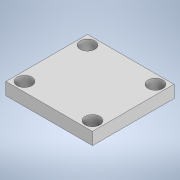
# Autodesk Inventor part: Phone Mount Cover V1
Saved by Autodesk Inventor 2020.2 (Build 242310000, 310)
## iProperties
Created: 2020-02-25
Part Number: Phone Mount Cover V1
Material: Generic
Document SubType Name: Modeling
Designer: AOFUser
Density: 1 g/cm^3
Appearance: Default
Author: AOFUser
Autodesk Inventor part; units mm, degrees
ref_plane "YZ Plane" through (0, 0, 0) normal (1, 0, 0) x (0, 1, 0)
ref_plane "XZ Plane" through (0, 0, 0) normal (0, 1, 0) x (-1, 0, 0)
ref_plane "XY Plane" through (0, 0, 0) normal (0, 0, 1) x (1, 0, 0)
sketch "Sketch1" plane through (0, 0, 0) normal (0, 1, 0) x (-1, 0, 0)
  line L0 (0, 0) -> (-17.78, 0)
  line L1 (-17.78, 0) -> (-17.78, -16.764)
  line L2 (-17.78, -16.764) -> (0, -16.764)
  line L3 (0, -16.764) -> (0, 0)
  dimension "d0" = 17.78
  dimension "d1" = 16.764
  constraints: 8 end point, 2 parallel, 1 horizontal, 1 perpendicular
  measures "d0" distance of L2.end L1.end
  measures "d1" distance of L1.end L0.end
extrude "Extrusion1" add sketch "Sketch1" along normal blind 2.54
sketch "Sketch2" plane through (0, 2.54, 0) normal (0, 1, 0) x (1, 0, 0)
  line L0 (0, 0) -> (17.78, 0) projected
  line L1 (0, 0) -> (3.81, 0)
  line L2 (3.81, 0) -> (3.81, 3.81)
  line L3 (3.81, 3.81) -> (0, 3.81)
  line L4 (0, 3.81) -> (0, 0)
  line L5 (17.78, 16.764) -> (0, 16.764) projected
  line L6 (0, 16.764) -> (3.81, 16.764)
  line L7 (3.81, 16.764) -> (3.81, 12.954)
  line L8 (3.81, 12.954) -> (0, 12.954)
  line L9 (0, 12.954) -> (0, 16.764)
  line L10 (17.7651, 0) -> (13.9551, 0)
  line L11 (13.9551, 0) -> (13.9551, 3.81)
  line L12 (13.9551, 3.81) -> (17.7651, 3.81)
  line L13 (17.7651, 3.81) -> (17.7651, 0)
  line L14 (17.78, 0) -> (17.78, 16.764) projected
  line L15 (17.78, 16.764) -> (13.97, 16.764)
  line L16 (13.97, 16.764) -> (13.97, 12.954)
  line L17 (13.97, 12.954) -> (17.78, 12.954)
  line L18 (17.78, 12.954) -> (17.78, 16.764)
  point P0 (1.905, 1.905)
  point P1 (15.875, 1.905)
  point P2 (15.875, 14.859)
  point P3 (1.905, 14.859)
  dimension "d4" = 3.81
  dimension "d5" = 3.81
  dimension "d6" = 3.81
  dimension "d7" = 3.81
  dimension "d8" = 3.81
  dimension "d9" = 3.81
  dimension "d10" = 3.81
  dimension "d11" = 3.81
  constraints: 32 end point, 8 parallel, 4 horizontal, 4 perpendicular, 1 point on line
  measures "d4" distance of L3.end L2.end
  measures "d5" distance of L2.end L1.end
  measures "d6" distance of L7.end L8.end
  measures "d7" distance of L6.end L7.end
  measures "d8" distance of L11.end L12.end
  measures "d9" distance of L10.end L11.end
  measures "d10" distance of L17.end L16.end
  measures "d11" distance of L16.end L15.end
hole "Hole1" at (1.905, 2.54, -1.905) at (15.875, 2.54, -1.905) at (15.875, 2.54, -14.859) at (1.905, 2.54, -14.859) direction (0, -1, 0) diameter 3.048 depth 10.16 tip angle 118
body "Solid1"
